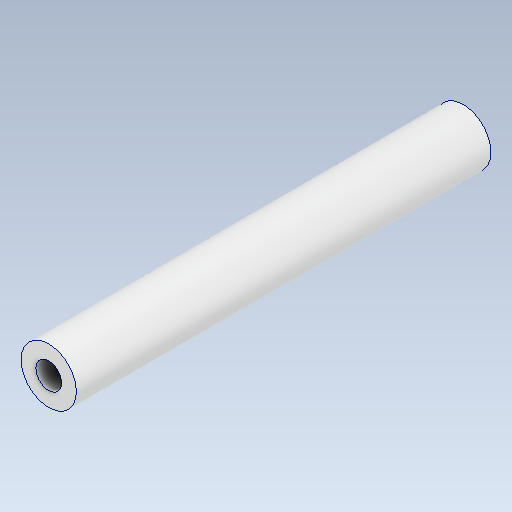
# Autodesk Inventor part: 40mm
Saved by Autodesk Inventor 2020 (Build 240168000, 168)
## iProperties
Created: 2020-02-27
Part Number: 40mm
Material: アルミニウム 6061
Document SubType Name: Modeling
Designer: happy
Density: 2.7 g/cm^3
Appearance: アルミニウム - フラット
Author: happy
Autodesk Inventor part; units mm, degrees
ref_plane "YZ Plane" through (0, 0, 0) normal (1, 0, 0) x (0, 1, 0)
ref_plane "XZ Plane" through (0, 0, 0) normal (0, 1, 0) x (-1, 0, 0)
ref_plane "XY Plane" through (0, 0, 0) normal (0, 0, 1) x (1, 0, 0)
sketch "スケッチ1" plane through (0, 0, 0) normal (0, 0, 1) x (1, 0, 0)
  circle A0 centre (0, 0) radius 1.4
  circle A1 centre (0, 0) radius 3
  dimension "d0" = 2.8
  dimension "d1" = 6
  constraints: 2 centre point, 2 coincident
  measures "d0" diameter of A0
  measures "d1" diameter of A1
extrude "押し出し1" add sketch "スケッチ1" along normal blind 45 contours A0 | A1
sketch "スケッチ2" plane through (0, 0, 45) normal (0, 0, 1) x (1, 0, 0)
  circle A0 centre (0, 0) radius 1.4
  dimension "d4" = 2.8
  constraints: 1 centre point, 1 coincident
  measures "d4" diameter of A0
extrude "押し出し2" cut sketch "スケッチ2" against normal blind 6
extrude "押し出し3" cut sketch "スケッチ1" along normal blind 6 contours A0
